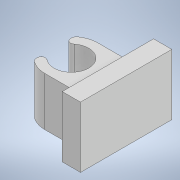
# Autodesk Inventor part: stand_mount_example
Saved by Autodesk Inventor 2020 (Build 240168000, 168)
## iProperties
Created: 2023-11-08
Part Number: stand_mount_example
Material: Типовые
Document SubType Name: Modeling
Designer: denis
Density: 1 g/cm^3
Appearance: По умолчанию
Author: denis
Autodesk Inventor part; units mm, degrees
ref_plane "YZ Plane" through (0, 0, 0) normal (1, 0, 0) x (0, 1, 0)
ref_plane "XZ Plane" through (0, 0, 0) normal (0, 1, 0) x (-1, 0, 0)
ref_plane "XY Plane" through (0, 0, 0) normal (0, 0, 1) x (1, 0, 0)
sketch "Эскиз1" plane through (0, 0, 0) normal (0, 1, 0) x (-1, 0, 0)
  line L0 (0, 25.8601) -> (0, -22.7313) construction
  arc A0 (8.1832, 2.5181) -> (8.1832, 6.1819) centre (6, 4.35) ccw construction
  line L1 (6, 4.35) -> (8.85, 4.35) construction
  line L2 (6, 4.35) -> (8.1832, 2.5181) construction
  line L3 (6, 4.35) -> (8.1832, 6.1819) construction
  arc A1 (6, 8.7) -> (6, 0) centre (6, 4.35) ccw construction
  line L4 (6, 0) -> (0, 0)
  line L5 (6, 8.7) -> (0, 8.7)
  arc A2 (9.3323, 7.1461) -> (6, 8.7) centre (6, 4.35) ccw
  arc A3 (9.3323, 1.5539) -> (9.3323, 7.1461) centre (6, 4.35) ccw construction
  arc A4 (6, 0) -> (9.3323, 1.5539) centre (6, 4.35) ccw
  line L6 (8.1832, 2.5181) -> (9.3323, 1.5539)
  line L7 (8.1832, 6.1819) -> (9.3323, 7.1461)
  arc A5 (8.1832, 6.1819) -> (8.1832, 2.5181) centre (6, 4.35) ccw
  line L8 (0, 0) -> (0, 8.7)
  line L9 (-3, 11.85) -> (0, 11.85)
  line L10 (0, 11.85) -> (0, -3.15)
  line L11 (0, -3.15) -> (-3, -3.15)
  line L12 (-3, -3.15) -> (-3, 11.85)
  point P0 (0, 4.35)
  point P1 (0, 0)
  point P2 (0, 8.7)
  dimension "d0" = 5.7
  dimension "d1" = 80
  dimension "d3" = 6
  dimension "d6" = 15
  dimension "d7" = 3
  dimension "d12" = 1.5
  dimension "d15" = 80
  constraints: 26 end point, 14 point on circle, 6 centre point, 6 tangent, 4 horizontal, 3 coincident, 3 point on line, 3 vertical, 2 midpoint, 2 parallel, 1 perpendicular, 1 symmetric about line, 1 other
  measures "d0" diameter of A0
  measures "d1" angle of L3 L2
  measures "d3" distance from line of L0 L1.start
  measures "d6" distance of L11.end L9.start
  measures "d7" distance of L10.end L11.end
  measures "d12" radial gap between concentric circles of A1 A5
  measures "d15" angle of L6 L7
extrude "Выдавливание1" add sketch "Эскиз1" along normal blind 8 contours L4 L8 L5 A2 L7 A5 L6 A4
extrude "Выдавливание2" add sketch "Эскиз1" along normal blind 10 contours L10 L11 L12 L9 L8
fillet "Сопряжение3" radius 0.7 2 edges at (-8.1832, 4, 2.5181) (-8.1832, 4, 6.1819)
fillet "Сопряжение4" radius 0.9 2 edges at (-9.3323, 4, 1.5539) (-9.3323, 4, 7.1461)
